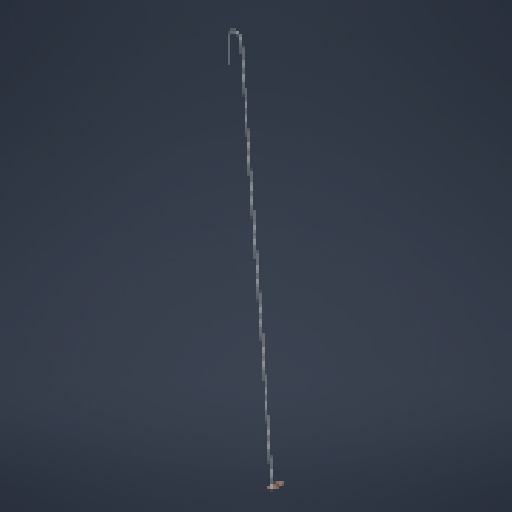
# Autodesk Inventor part: Rope
Saved by Autodesk Inventor 2023.6 (Build 276521000, 521)
## iProperties
Created: 2026-03-05
Part Number: Rope
Material: Generic
Document SubType Name: Modeling
Designer: user
Density: 1 g/cm^3
Appearance: Default
Author: user
Autodesk Inventor part; units mm, degrees
ref_plane "YZ Plane" through (0, 0, 0) normal (1, 0, 0) x (0, 1, 0)
ref_plane "XZ Plane" through (0, 0, 0) normal (0, 1, 0) x (-1, 0, 0)
ref_plane "XY Plane" through (0, 0, 0) normal (0, 0, 1) x (1, 0, 0)
sketch "Sketch1" plane through (0, 0, 0) normal (0, 0, 1) x (1, 0, 0)
  line L0 (33.5736, -359.3435) -> (37.5586, -358.9974) projected
  circle A0 centre (0, 0) radius 5 projected
  arc A1 (5.4809, 0.4585) -> (-5.5, 0) centre (0, 0) ccw
  line L1 (35.5661, -359.1705) -> (5.4809, 0.4585)
  line L2 (-5.5, 0) -> (-5.5, -25)
  dimension "d0" = 11
  dimension "d1" = 25
  dimension "d2" = 360.8852
  constraints: 4 end point, 2 point on circle, 2 tangent, 1 centre point, 1 coincident, 1 midpoint, 1 vertical
  measures "d0" diameter of A1
  measures "d1" distance of L2.start L2.end
  measures "d2" distance of L1.start L1.end
ref_plane "Work Plane1" through (33.5736, -359.3435, -9) normal (-0.0865, 0.9962, 0) x (-0.9962, -0.0865, 0)
sketch "Sketch2" plane through (33.5736, -359.3435, -9) normal (-0.0865, 0.9962, 0) x (-0.9962, -0.0865, 0)
  circle A0 centre (-2, 9) radius 0.5 projected
  circle A1 centre (-2, 9) radius 0.5
  point P0 (2.3507, 9)
  constraints: 1 centre point, 1 coincident, 1 concentric
sweep "Sweep1" add profiles "Sketch2" path "Sketch1" path curves L1 A1
body "Solid1"
